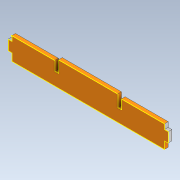
# Autodesk Inventor part: chassis_1_6
Saved by Autodesk Inventor 2022 (Build 260153000, 153)
## iProperties
Created: 2023-04-28
Part Number: chassis_1_6
Material: 一般
Document SubType Name: Modeling
Designer: Johnny Jou
Density: 1 g/cm^3
Appearance: 預設
Author: Johnny Jou
Autodesk Inventor part; units mm, degrees
ref_plane "YZ Plane" through (0, 0, 0) normal (1, 0, 0) x (0, 1, 0)
ref_plane "XZ Plane" through (0, 0, 0) normal (0, 1, 0) x (-1, 0, 0)
ref_plane "XY Plane" through (0, 0, 0) normal (0, 0, 1) x (1, 0, 0)
sketch "草圖1" plane through (0, 0, 0) normal (0, 0, 1) x (1, 0, 0)
  line L0 (0, 0) -> (124, 0)
  line L1 (124, 0) -> (124, -18) construction
  line L2 (124, -18) -> (0, -18)
  line L3 (0, -18) -> (0, 0) construction
  line L4 (35, 0) -> (37.95, 0)
  line L5 (37.95, 0) -> (37.95, -7.5)
  line L6 (37.95, -7.5) -> (35, -7.5)
  line L7 (35, -7.5) -> (35, 0)
  line L8 (89, 0) -> (86.05, 0)
  line L9 (86.05, 0) -> (86.05, -7.5)
  line L10 (86.05, -7.5) -> (89, -7.5)
  line L11 (89, -7.5) -> (89, 0)
  line L12 (0, -18) -> (0, 0) construction
  line L13 (-3, -12) -> (0, -12)
  line L14 (0, -12) -> (0, -18)
  line L15 (124, -12) -> (124, -18)
  line L16 (-3, -12) -> (-3, -4)
  line L17 (-3, -4) -> (0, -4)
  line L18 (0, 0) -> (0, -4)
  line L19 (124, -12) -> (127, -12)
  line L20 (127, -12) -> (127, -4)
  line L21 (127, -4) -> (124, -4)
  line L22 (124, -4) -> (124, -12)
  line L23 (124, 0) -> (124, -4)
  point P0 (0, -15.5)
  dimension "d0" = 124
  dimension "d1" = 35
  dimension "d3" = 2.95
  dimension "d4" = 2.95
  dimension "d10" = 10.5
  dimension "d16" = 7.5
  dimension "d17" = 35
  dimension "d29" = 8
  dimension "d30" = 4
  dimension "d31" = 3
  dimension "d32" = 3
  dimension "d33" = 4
  dimension "d34" = 8
  constraints: 48 end point, 8 parallel, 6 perpendicular, 5 point on line, 4 horizontal, 2 collinear, 1 vertical
  measures "d0" distance of L1.end L2.end
  measures "d1" distance between parallel lines of L3 L7
  measures "d3" distance of L5.end L6.end
  measures "d4" distance of L9.end L10.end
  measures "d10" distance between parallel lines of L2 L6
  measures "d16" distance of L6.end L4.start
  measures "d17" distance between parallel lines of L1 L11
  measures "d29" distance of L13.start L16.end
  measures "d30" distance between parallel lines of L0 L17
  measures "d31" distance between parallel lines of L3 L16
  measures "d32" distance between parallel lines of L1 L20
  measures "d33" distance between parallel lines of L0 L21
  measures "d34" distance between parallel lines of L19 L21
extrude "擠出1" add sketch "草圖1" along normal blind 3 contours L0 L7 L6 L5 L9 L10 L11 L23 L22 L15 L2 L14 L13 L16 L17 L18 | L21 L20 L19 L22
sketch "草圖2" plane through (0, 0, 3) normal (0, 0, 1) x (1, 0, 0)
  line L0 (37.95, 0) -> (86.05, 0)
  line L1 (86.05, 0) -> (86.05, 2)
  line L2 (86.05, 2) -> (37.95, 2)
  line L3 (37.95, 2) -> (37.95, 0)
  line L4 (86.05, -7.5) -> (86.05, 0) projected
  point P0 (0, 0)
  dimension "d26" = 2
  constraints: 8 end point, 2 parallel, 1 collinear, 1 horizontal, 1 perpendicular
  measures "d26" distance between parallel lines of L0 L2
extrude "擠出2" add sketch "草圖2" against normal up to surface (3 mm away)
sketch "草圖3" plane through (0, 0, 3) normal (0, 0, 1) x (1, 0, 0)
  line L0 (124, 0) -> (89, 0) projected
  line L1 (89, 0) -> (89, -7.5) projected
  line L2 (89, -7.5) -> (86.05, -7.5) projected
  line L3 (86.05, -7.5) -> (86.05, 2) projected
  line L4 (37.95, -7.5) -> (35, -7.5) projected
  line L5 (35, -7.5) -> (35, 0) projected
  line L6 (35, 0) -> (0, 0) projected
  line L7 (0, -4) -> (-3, -4) projected
  line L8 (-3, -4) -> (-3, -12) projected
  line L9 (-3, -12) -> (0, -12) projected
  line L10 (0, -12) -> (0, -18) projected
  line L11 (0, -18) -> (124, -18) projected
  line L12 (124, -18) -> (124, -12) projected
  line L13 (124, -12) -> (127, -12) projected
  line L14 (127, -12) -> (127, -4) projected
  line L15 (127, -4) -> (124, -4) projected
  line L16 (124, -4) -> (124, 0) projected
  line L17 (86.05, 2) -> (37.95, 2) projected
  line L18 (37.95, 2) -> (37.95, -7.5) projected
  line L19 (0, 0) -> (0, -4) projected
